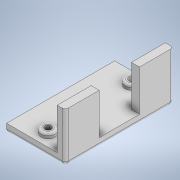
# Autodesk Inventor part: springBedMount
Saved by Autodesk Inventor 2020 (Build 240168000, 168)
## iProperties
Created: 2020-07-27
Part Number: springBedMount
Material: Generic
Document SubType Name: Modeling
Designer: PAB
Density: 1 g/cm^3
Appearance: Default
Author: PAB
Autodesk Inventor part; units mm, degrees
ref_plane "YZ Plane" through (0, 0, 0) normal (1, 0, 0) x (0, 1, 0)
ref_plane "XZ Plane" through (0, 0, 0) normal (0, 1, 0) x (-1, 0, 0)
ref_plane "XY Plane" through (0, 0, 0) normal (0, 0, 1) x (1, 0, 0)
sketch "Sketch1" plane through (0, 0, 0) normal (0, 1, 0) x (-1, 0, 0)
  line L0 (18.7, 33.5) -> (-17.7, 33.5)
  line L1 (-17.7, 33.5) -> (-17.7, -33.5)
  line L2 (-17.7, -33.5) -> (18.7, -33.5)
  line L3 (18.7, -33.5) -> (18.7, 33.5)
  point P0 (0, 0)
  dimension "d0" = 36.4
  dimension "d1" = 67
  constraints: 8 end point, 2 parallel, 1 horizontal, 1 perpendicular
  measures "d0" distance of L2.end L1.end
  measures "d1" distance of L1.end L0.end
extrude "Extrusion1" add sketch "Sketch1" along normal blind 5
sketch "Sketch2" plane through (0, 5, 0) normal (0, 1, 0) x (1, 0, 0)
  line L0 (-18.7, -33.5) -> (17.7, -33.5) projected
  line L1 (17.7, -33.5) -> (12.7, -33.5)
  line L2 (12.7, -33.5) -> (12.7, -12.5)
  line L3 (12.7, -12.5) -> (17.7, -12.5)
  line L4 (17.7, -12.5) -> (17.7, -33.5)
  line L5 (17.7, -33.5) -> (17.7, 33.5) projected
  line L6 (17.7, 33.5) -> (12.7, 33.5)
  line L7 (12.7, 33.5) -> (12.7, 12.5)
  line L8 (12.7, 12.5) -> (17.7, 12.5)
  line L9 (17.7, 12.5) -> (17.7, 33.5)
  point P0 (0, 0)
  dimension "d4" = 5
  dimension "d5" = 21
  dimension "d6" = 5
  dimension "d7" = 21
  constraints: 16 end point, 4 parallel, 2 horizontal, 2 perpendicular
  measures "d4" distance of L2.end L3.end
  measures "d5" distance of L1.end L2.end
  measures "d6" distance of L8.end L7.end
  measures "d7" distance of L7.end L6.end
extrude "Extrusion2" add sketch "Sketch2" along normal blind 25.4
sketch "Sketch3" plane through (0, 5, 0) normal (0, 1, 0) x (1, 0, 0)
  circle A0 centre (-0.5, -26) radius 4.25
  circle A1 centre (0, 0) radius 4.25
  circle A2 centre (-0.5, 26) radius 4.25
  line L0 (-18.7, 33.5) -> (-18.7, -33.5) projected
  dimension "d10" = 8.5
  dimension "d11" = 8.5
  dimension "d12" = 8.5
  dimension "d26" = 18.2
  dimension "d27" = 18.2
  constraints: 3 centre point, 1 coincident
  measures "d10" diameter of A0
  measures "d11" diameter of A1
  measures "d12" diameter of A2
  measures "d26" distance from line of L0 A2.centre
  measures "d27" distance from line of L0 A0.centre
extrude "Extrusion3" add sketch "Sketch3" along normal blind 3 contours A0 | A2
sketch "Sketch4" plane through (0, 0, 0) normal (0, -1, 0) x (1, 0, 0)
  circle A0 centre (-0.5, -26) radius 4.25 projected
  circle A1 centre (-0.5, -26) radius 3
  circle A2 centre (-0.5, 26) radius 4.25 projected
  circle A3 centre (-0.5, 26) radius 3
  point P0 (0, 0)
  dimension "d15" = 6
  dimension "d16" = 6
  constraints: 2 centre point, 2 coincident
  measures "d15" diameter of A1
  measures "d16" diameter of A3
extrude "Extrusion4" cut sketch "Sketch4" against normal blind 3 contours A1 | A3
sketch "Sketch5" plane through (0, 0, 0) normal (0, -1, 0) x (1, 0, 0)
  circle A0 centre (-0.5, -26) radius 3 projected
  circle A1 centre (-0.5, -26) radius 2
  circle A2 centre (-0.5, 26) radius 4.25 projected
  circle A3 centre (-0.5, 26) radius 2
  circle A4 centre (-0.5, 0) radius 2
  point P0 (0, 0)
  dimension "d19" = 4
  dimension "d21" = 4
  dimension "d30" = 4
  constraints: 3 centre point, 2 coincident
  measures "d19" diameter of A1
  measures "d21" diameter of A3
  measures "d30" diameter of A4
extrude "Extrusion5" cut sketch "Sketch5" against normal blind 15 contours A1 | A3 | A4
fillet "Fillet1" radius 1.5 2 edges at (-4.75, 8, 26) (-4.75, 8, -26)
fillet "Fillet2" radius 2 6 edges at (-0.5, 0, 33.5) (-18.7, 0, 0) (17.7, 15.2, 33.5) (17.7, 15.2, -33.5) (-0.5, 0, -33.5) (17.7, 0, 0)
body "Solid1"
